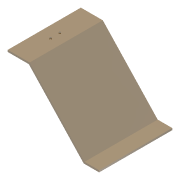
# Autodesk Inventor part: ramp
Saved by Autodesk Inventor 2015 (Build 190159000, 159)
## iProperties
Created: 2015-01-25
Part Number: ramp
Material: Generic
Document SubType Name: Modeling
Designer: rihoobler
Density: 1 g/cm^3
Appearance: Polycarbonate - Smoked
Author: rihoobler
Autodesk Inventor part; units mm, degrees
ref_plane "YZ Plane" through (0, 0, 0) normal (1, 0, 0) x (0, 1, 0)
ref_plane "XZ Plane" through (0, 0, 0) normal (0, 1, 0) x (-1, 0, 0)
ref_plane "XY Plane" through (0, 0, 0) normal (0, 0, 1) x (1, 0, 0)
sketch "Sketch1" plane through (0, 0, 0) normal (0, 0, 1) x (1, 0, 0)
  line L0 (0, 0) -> (38.1, 0)
  line L1 (158.7411, -101.6561) -> (133.3411, -101.6561)
  line L2 (158.7411, -101.6561) -> (184.1411, -101.6561) construction
  line L3 (133.3411, -101.6561) -> (38.1, 0)
  line L4 (0, -3.175) -> (36.7239, -3.175)
  line L5 (36.7239, -3.175) -> (131.965, -104.8311)
  line L6 (131.965, -104.8311) -> (158.7411, -104.8311)
  line L7 (158.7411, -104.8311) -> (184.15, -104.8311)
  line L8 (0, 0) -> (0, -3.175)
  line L9 (158.7411, -101.6561) -> (158.7411, -104.8311)
  dimension "d2" = 38.1
  dimension "d3" = 25.4
  dimension "d4" = 180
  dimension "d5" = 3.175
  constraints: 20 end point, 2 horizontal, 1 collinear, 1 parallel, 1 vertical, 3 other
  measures "d2" distance of L0.start L0.end
  measures "d3" distance of L1.start L1.end
  measures "d4" angle of L1 L2
  measures "d5" distance between parallel lines of L0 L4
extrude "Extrusion1" add sketch "Sketch1" along normal blind 127
sketch "Sketch2" plane through (0, 0, 0) normal (0, 1, 0) x (1, 0, 0)
  line L0 (0, 0) -> (38.1, 0) projected
  line L1 (0, 0) -> (0, -127) projected
  point P0 (19.05, -55.5)
  point P1 (19.05, -71.5)
  dimension "d8" = 16
  dimension "d10" = 55.5
  dimension "d11" = 19.05
  measures "d8" distance of point (19.05, -55.5) point (19.05, -71.5)
  measures "d10" distance from line of L0 point (19.05, -55.5)
  measures "d11" distance from line of L1 point (19.05, -55.5)
hole "Hole1" at (19.05, 0, 55.5) at (19.05, 0, 71.5) direction (0, -1, 0) diameter 3.175 end through all
body "Solid1"
